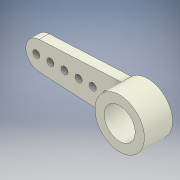
# Autodesk Inventor part: orczyk_1_2
Saved by Autodesk Inventor 2018 (Build 220112000, 112)
## iProperties
Created: 2020-10-02
Part Number: orczyk_1_2
Material: Ogólny
Document SubType Name: Modeling
Designer: Raven
Density: 1 g/cm^3
Appearance: Domyślna
Author: Raven
Autodesk Inventor part; units mm, degrees
ref_plane "YZ Plane" through (0, 0, 0) normal (1, 0, 0) x (0, 1, 0)
ref_plane "XZ Plane" through (0, 0, 0) normal (0, 1, 0) x (-1, 0, 0)
ref_plane "XY Plane" through (0, 0, 0) normal (0, 0, 1) x (1, 0, 0)
sketch "Szkic1" plane through (0, 0, 0) normal (0, 1, 0) x (-1, 0, 0)
  circle A0 centre (0, 0) radius 3.5 construction
  line L0 (-3.5, 0.0079) -> (15.9, 0.0079) construction
  line L1 (15.9, 0.0079) -> (13.9, 0.0079) construction
  circle A1 centre (13.9, 0.0079) radius 2 construction
  line L2 (2.3431, 2.6) -> (2.3431, -2.6) construction
  line L3 (14.0019, 2.0053) -> (2.3431, 2.6) construction
  line L4 (14.0019, -1.9895) -> (2.3431, -2.6) construction
  circle A2 centre (0, 0) radius 2.2
  arc A3 (14.0019, -1.9895) -> (14.0019, 2.0053) centre (13.9, 0.0079) ccw
  arc A4 (2.3431, 2.6) -> (2.3431, -2.6) centre (0, 0) ccw
  line L5 (14.0019, 2.0053) -> (2.3431, 2.6)
  line L6 (2.3431, -2.6) -> (14.0019, -1.9895)
  dimension "d0" = 7
  dimension "d1" = 19.4
  dimension "d2" = 3.5
  dimension "d3" = 2
  dimension "d4" = 5.2
  dimension "d5" = 4.4
  dimension "d24" = 11.6588
  dimension "d25" = 11.6588
  constraints: 14 end point, 12 point on circle, 5 centre point, 3 coincident, 1 collinear, 1 horizontal, 1 perpendicular, 1 point on line, 1 tangent
  measures "d0" diameter of A0
  measures "d1" distance of L0.start L0.end
  measures "d2" distance of L0.start point (0, 0)
  measures "d3" distance of L0.end L1.end
  measures "d4" distance of L2.start L2.end
  measures "d5" diameter of A2
  measures "d24" horizontal distance of L3.start L2.start
  measures "d25" horizontal distance of L4.start L2.end
extrude "Wyciągnięcie proste1" add sketch "Szkic1" along normal blind 1.4
sketch "Szkic2" plane through (0, 0, 0) normal (0, -1, 0) x (1, 0, 0)
  circle A0 centre (0, 0) radius 3.5
  circle A1 centre (0, 0) radius 2.2
  constraints: 2 centre point, 2 coincident
extrude "Wyciągnięcie proste2" add sketch "Szkic2" along normal blind 2.6
sketch "Szkic3" plane through (0, 1.4, 0) normal (0, 1, 0) x (1, 0, 0)
  circle A0 centre (0, 0) radius 2.2 construction
  line L0 (-2.2, -0.0079) -> (-15.9, -0.0079) construction
  arc A1 (-14.0019, 1.9895) -> (-14.0019, -2.0053) centre (-13.9, -0.0079) ccw construction
  line L1 (-15.9, -0.0079) -> (-14.4, -0.0079) construction
  circle A2 centre (-14.4, -0.0079) radius 0.5
  line L2 (-14.4, -0.0079) -> (-12.4, -0.0079) construction
  line L3 (-12.4, -0.0079) -> (-10.4, -0.0079) construction
  line L4 (-10.4, -0.0079) -> (-8.4, -0.0079) construction
  line L5 (-8.4, -0.0079) -> (-6.4, -0.0079) construction
  line L6 (-6.4, -0.0079) -> (-4.4, -0.0079) construction
  circle A3 centre (-12.4, -0.0079) radius 0.5
  circle A4 centre (-10.4, -0.0079) radius 0.5
  circle A5 centre (-8.4, -0.0079) radius 0.5
  circle A6 centre (-6.4, -0.0079) radius 0.5
  circle A7 centre (-4.4, -0.0079) radius 0.5
  point P0 (0, 0)
  dimension "d10" = 1.5
  dimension "d11" = 1
  dimension "d12" = 2
  dimension "d13" = 2
  dimension "d14" = 2
  dimension "d15" = 2
  dimension "d16" = 2
  dimension "d17" = 1
  dimension "d18" = 1
  dimension "d19" = 1
  dimension "d20" = 1
  dimension "d21" = 1
  constraints: 14 end point, 6 centre point, 6 coincident, 6 point on line, 1 horizontal, 1 point on circle, 2 other
  measures "d10" distance of L0.end L1.end
  measures "d11" diameter of A2
  measures "d12" distance of L2.start L2.end
  measures "d13" distance of L2.end L3.end
  measures "d14" distance of L3.end L4.end
  measures "d15" distance of L4.end L5.end
  measures "d16" distance of L5.end L6.end
  measures "d17" diameter of A3
  measures "d18" diameter of A4
  measures "d19" diameter of A5
  measures "d20" diameter of A6
  measures "d21" diameter of A7
extrude "Wyciągnięcie proste3" cut sketch "Szkic3" against normal blind 1.4
equation "\"d25\" = d24"
